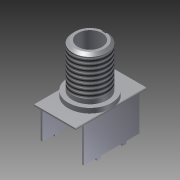
# Autodesk Inventor part: M201S1M201-bushing
Saved by Autodesk Inventor 2014 (Build 180170000, 170)
## iProperties
Category: PARTsolutions
Company: NKKSWITCHES
Created: 2013-12-29
Part Number: M201S1M201-bushing
Catalog Web Link: www.cadenas.de
Description: Bushing Mount Miniature Toggles - Bushing-Series M - Miniature Toggles
Vendor: NKKSWITCHES
Document SubType Name: Modeling
Designer: PARTuser1
Manufacturer: NKKSWITCHES
Density: 1 g/cm^3
Material: Generic
Appearance: RGB(192.00000375509219,192.00000375509219,192.00000375509219)
PSOL_IDENT_0: {$CADENAS_DATA\23d-libs\nkkswitches\toggle\m\parts\m_bt_cover.prj},222 {VTYP=3D},{NB=M201S1M201-bush
PSOL_IDENT_1: ing},{LINA=M201S1M201-bushing},{NN=Bushing Mount Miniature Toggles - Bushing},{DATE=28.05.2013 11:17
PSOL_IDENT_2: :51},{GEOMDATE=28.05.2013 13:17:00},{VERSION=},{LINEID=10},{LINESUBID=-1},{WBVAR=PLS,BSHNG}  {NB=M20
PSOL_IDENT_3: 1S1M201-bushing},{LINA=M201S1M201-bushing},{KT=DUMMY},{PN=M201S1M201},{SRS=M20},{PLS=1},{BSHNGALG='S
PSOL_IDENT_4: 1', 'S1 - .350\" (8.9mm) Threaded with Keyway','S2', 'S2 - .350\" (8.9mm) Smooth with Keyway','A1',
PSOL_IDENT_5: 'A1 - .280\" (7.1mm) Threaded with Keyway','A2', 'A2 - .280\" (7.1mm) Smooth with Keyway','D1', 'D1
PSOL_IDENT_6: - .350\" (8.9mm) Threaded with D Flat','D4' , 'D4 - 6mm .350\" (8.9mm) Threaded with D Flat ' ,'D3',
PSOL_IDENT_7: 'D3 - .350\" (8.9mm) Threaded Splashproof with D Flat','S4', 'S4 - 6mm .350\" (8.9mm) Threaded with
PSOL_IDENT_8: Keyway','D8', 'D8 - .350\" (8.9mm) 6mm Threaded Splashproof with D Flat','B1', 'B1 - Large .472\" (
PSOL_IDENT_9: 12mm) Threaded with Keyway','B3', 'B3 - Large .472\" (12mm) Threaded Splashproof with D Flat','L1',
PSOL_IDENT_10: 'L1 - .291\" (7.4mm) Threaded with Keyway for Lever Lock','L4' , 'L4 - 6mm .291\" (7.4mm) Threaded w
PSOL_IDENT_11: ith Keyway for Lever Lock' ,'L2', 'L2 - Smooth with Keyway for Lever Lock','L3', 'L3 - .295\" (7.5mm
PSOL_IDENT_12: ) Threaded Splashproof with D Flat for Lever Lock','L8' , 'L8 - 6mm .295\" (7.5mm) Threaded Splashpr
PSOL_IDENT_13: oof with D Flat for Lever Lock'},{BSHNG=S1},{WIDTH=0.512},{HEIGHT=0.37},{LENGTH=0.311},{A=0},{TRMNLN
PSOL_IDENT_14: OH=1},{DMAJ=0.25},{DMIN=0.2193},{BSHNGDIA=0.315},{THRDL=0.35},{THRDL2=0.035},{PCDIA=0.256},{PC2=0.22
PSOL_IDENT_15: },{PC3=0.024},{KEYPOS=0.098},{KEYW=0.031}
CNS_NN: Bushing Mount Miniature Toggles - Bushing
CNS_NT: Series M - Miniature Toggles
CNS_NB: M201S1M201-bushing
CNS_NBSYN: $PN.-bushing
CNS_LINA: M201S1M201-bushing
CNS_PN: M201S1M201
CNS_SRS: M20
CNS_PLS: 1 - SPST/SPDT
CNS_BSHNGALG: 'S1', 'S1 - .350" (8.9mm) Threaded with Keyway','S2', 'S2 - .350" (8.9mm) Smooth with Keyway','A1', 'A1 - .280" (7.1mm) Threaded with Keyway','A2', 'A2 - .280" (7.1mm) Smooth with Keyway','D1', 'D1 - .350" (8.9mm) Threaded with D Flat','D4' , 'D4 - 6mm .350" (8.9mm) Threaded with D Flat ' ,'D3', 'D3 - .350" (8.9mm) Threaded Splashproof with D Flat','S4', 'S4 - 6mm .350" (8.9mm) Threaded with Keyway','D8', 'D8 - .350" (8.9mm) 6mm Threaded Splashproof with D Flat','B1', 'B1 - Large .472" (12mm) Threaded with Keyway','B3', 'B3 - Large .472" (12mm) Threaded Splashproof with D Flat','L1', 'L1 - .291" (7.4mm) Threaded with Keyway for Lever Lock','L4' , 'L4 - 6mm .291" (7.4mm) Threaded with Keyway for Lever Lock' ,'L2', 'L2 - Smooth with Keyway for Lever Lock','L3', 'L3 - .295" (7.5mm) Threaded Splashproof with D Flat for Lever Lock','L8' , 'L8 - 6mm .295" (7.5mm) Threaded Splashproof with D Flat for Lever Lock'
CNS_BSHNG: S1 - .350" (8.9mm) Threaded with Keyway
CNS_WIDTH: 0.512
CNS_HEIGHT: 0.370
CNS_LENGTH: 0.311
CNS_A: 0.000
CNS_TRMNLNOH: 1.000
CNS_DMAJ: 0.250
CNS_DMIN: 0.219
CNS_BSHNGDIA: 0.315
CNS_THRDL: 0.350
CNS_THRDL2: 0.035
CNS_PCDIA: 0.256
CNS_PC2: 0.220
CNS_PC3: 0.024
CNS_KEYPOS: 0.098
CNS_KEYW: 0.031
SUPPLIER: NKKSWITCHES
ARTICLENO: M201S1M201-bushing
BOMINFO: M201S1M201-bushing
CREATOR: CADENAS GmbH
Title: M201S1M201-bushing
Author: Cadenas PARTsolutions
Comments: Series M - Miniature Toggles
Autodesk Inventor part; units mm, degrees
sketch "Sketch_1" plane through (0, 0, 0) normal (0, 0, 1) x (1, 0, 0)
  line L0 (-3.9497, 0) -> (-3.9497, -6.7945)
  line L1 (-3.9497, -6.7945) -> (-3.6957, -6.7945)
  line L2 (-3.6957, -6.7945) -> (-3.6957, -0.254)
  arc A0 (-3.4417, 0) -> (-3.6957, -0.254) centre (-3.4417, -0.254) ccw
  line L3 (-3.4417, 0) -> (3.4417, 0)
  arc A1 (3.6957, -0.254) -> (3.4417, 0) centre (3.4417, -0.254) ccw
  line L4 (3.6957, -0.254) -> (3.6957, -6.7945)
  line L5 (3.6957, -6.7945) -> (3.9497, -6.7945)
  line L6 (3.9497, -6.7945) -> (3.9497, 0)
  arc A2 (3.9497, 0) -> (3.6957, 0.254) centre (3.6957, 0) ccw
  line L7 (3.6957, 0.254) -> (-3.6957, 0.254)
  arc A3 (-3.6957, 0.254) -> (-3.9497, 0) centre (-3.6957, 0) ccw
  constraints: 16 end point, 8 point on circle, 4 centre point
extrude "Extrusion1" add sketch "Sketch_1" along normal mid plane 13.0048
sketch "Sketch_2" plane through (0, 0, 0) normal (1, 0, 0) x (0, 1, 0)
  line L0 (0, 7.8029) -> (-9.398, 7.8029)
  line L1 (-9.398, 7.8029) -> (-9.398, -7.8029)
  line L2 (-9.398, -7.8029) -> (0, -7.8029)
  line L3 (0, -7.8029) -> (0, -5.0927)
  line L4 (0, -5.0927) -> (-6.3246, -5.0927)
  line L5 (-6.3246, -5.0927) -> (-6.3246, -2.7305)
  line L6 (-6.3246, -2.7305) -> (-6.6675, -2.7305)
  arc A0 (-6.7945, -2.6035) -> (-6.6675, -2.7305) centre (-6.6675, -2.6035) ccw
  line L7 (-6.7945, -2.6035) -> (-6.7945, -2.0955)
  arc A1 (-6.6675, -1.9685) -> (-6.7945, -2.0955) centre (-6.6675, -2.0955) ccw
  line L8 (-6.6675, -1.9685) -> (-6.3246, -1.9685)
  line L9 (-6.3246, -1.9685) -> (-6.3246, 1.9685)
  line L10 (-6.3246, 1.9685) -> (-6.6675, 1.9685)
  arc A2 (-6.7945, 2.0955) -> (-6.6675, 1.9685) centre (-6.6675, 2.0955) ccw
  line L11 (-6.7945, 2.0955) -> (-6.7945, 2.6035)
  arc A3 (-6.6675, 2.7305) -> (-6.7945, 2.6035) centre (-6.6675, 2.6035) ccw
  line L12 (-6.6675, 2.7305) -> (-6.3246, 2.7305)
  line L13 (-6.3246, 2.7305) -> (-6.3246, 5.0927)
  line L14 (-6.3246, 5.0927) -> (0, 5.0927)
  line L15 (0, 5.0927) -> (0, 7.8029)
  constraints: 32 end point, 8 point on circle, 4 centre point
extrude "Extrusion2" cut sketch "Sketch_2" along normal mid plane 7.8994
sketch "Sketch_15" plane through (0, 0, 0) normal (0, 0, 1) x (1, 0, 0)
  line L0 (0, 0.127) -> (0, 9.144)
  line L1 (0, 9.144) -> (2.7026, 9.144)
  line L2 (2.7026, 9.144) -> (3.175, 8.6716)
  line L3 (3.175, 8.6716) -> (3.175, 1.143)
  line L4 (3.175, 1.143) -> (4.0005, 1.143)
  line L5 (4.0005, 1.143) -> (4.0005, 0.254)
  line L6 (4.0005, 0.254) -> (2.2225, 0.254)
  line L7 (2.2225, 0.254) -> (2.2225, 0.127)
  line L8 (2.2225, 0.127) -> (0, 0.127)
  line L9 (0, 0.127) -> (0, 9.144)
  constraints: 20 end point
revolve "Revolution1" add sketch "Sketch_15" angle 360 about axis through (0, 0.127, 0) along (0, -1, 0)
thread "Thread1" size "1/4-32 UNEF" class "2A" standard "ANSI Unified Screw Threads" length 7.239 offset 0.762
sketch "Sketch_8" plane through (0, 0.254, 0) normal (0, 1, 0) x (1, 0, 0)
  line L0 (-0.3937, 2.4892) -> (0.3937, 2.4892)
  line L1 (0.3937, 2.4892) -> (0.3937, 10.4902)
  line L2 (0.3937, 10.4902) -> (-0.3937, 10.4902)
  line L3 (-0.3937, 10.4902) -> (-0.3937, 2.4892)
  constraints: 8 end point
extrude "Extrusion3" cut sketch "Sketch_8" along normal blind 9.779
sketch "Sketch5" plane through (-3.9497, 0, -6.5024) normal (0, -1, 0) x (1, 0, 0)
  point P0 (3.9497, 6.5024)
hole "Drilling 1" at (0, 0, 0) direction (0, 1, 0) diameter 4.445 depth 9.144
ref_plane "1_XY" through (0, 7.112, 0) normal (0, 1, 0) x (1, 0, 0)
ref_plane "1_YZ" through (0, 7.112, 0) normal (1, 0, 0) x (0, 0, -1)
ref_plane "1_ZX" through (0, 7.112, 0) normal (0, 0, -1) x (0, 1, 0)
ref_plane "2_XY" through (0, 5.334, 0) normal (0, 1, 0) x (1, 0, 0)
ref_plane "2_YZ" through (0, 5.334, 0) normal (1, 0, 0) x (0, 0, -1)
ref_plane "2_ZX" through (0, 5.334, 0) normal (0, 0, -1) x (0, 1, 0)
ref_plane "3_XY" through (0, 3.556, 0) normal (0, 1, 0) x (1, 0, 0)
ref_plane "3_YZ" through (0, 3.556, 0) normal (1, 0, 0) x (0, 0, -1)
ref_plane "3_ZX" through (0, 3.556, 0) normal (0, 0, -1) x (0, 1, 0)
ref_plane "4_XY" through (0, 2.2225, 0) normal (0, 1, 0) x (1, 0, 0)
ref_plane "4_YZ" through (0, 2.2225, 0) normal (1, 0, 0) x (0, 0, -1)
ref_plane "4_ZX" through (0, 2.2225, 0) normal (0, 0, -1) x (0, 1, 0)
ref_plane "to_base_XY" through (0, 0, 0) normal (0, 1, 0) x (1, 0, 0)
ref_plane "to_base_YZ" through (0, 0, 0) normal (1, 0, 0) x (0, 0, -1)
ref_plane "to_base_ZX" through (0, 0, 0) normal (0, 0, -1) x (0, 1, 0)
body "Solid1"
